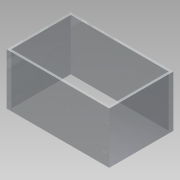
# Autodesk Inventor part: glass tank
Saved by Autodesk Inventor 2015 (Build 190159000, 159)
## iProperties
Created: 2015-05-21
Part Number: glass tank
Material: Glass
Document SubType Name: Modeling
Designer: Joe Sheldon
Density: 2.18 g/cm^3
Appearance: Clear
Author: Joe Sheldon
Autodesk Inventor part; units mm, degrees
ref_plane "YZ Plane" through (0, 0, 0) normal (1, 0, 0) x (0, 1, 0)
ref_plane "XZ Plane" through (0, 0, 0) normal (0, 1, 0) x (-1, 0, 0)
ref_plane "XY Plane" through (0, 0, 0) normal (0, 0, 1) x (1, 0, 0)
sketch "Sketch1" plane through (0, 0, 0) normal (0, 1, 0) x (-1, 0, 0)
  line L0 (0, 0) -> (406.4, 0)
  line L1 (406.4, 0) -> (406.4, -254)
  line L2 (406.4, -254) -> (0, -254)
  line L3 (0, -254) -> (0, 0)
  line L4 (396.875, -244.475) -> (396.875, -9.525)
  line L5 (396.875, -9.525) -> (9.525, -9.525)
  line L6 (9.525, -9.525) -> (9.525, -244.475)
  line L7 (9.525, -244.475) -> (396.875, -244.475)
  dimension "d0" = 406.4
  dimension "d1" = 254
  dimension "d2" = 9.525
  constraints: 16 end point, 4 parallel, 2 perpendicular, 1 horizontal, 3 other
  measures "d0" distance of L1.end L2.end
  measures "d1" distance of L0.end L1.end
  measures "d2" distance between parallel lines of L1 L4
extrude "Extrusion1" add sketch "Sketch1" along normal blind 203.2
body "Solid1"
